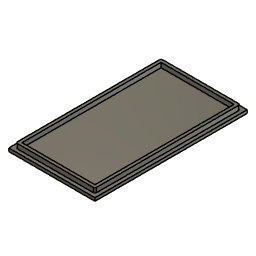
Tapa4_Base Final (Autodesk Fusion 360 design; units mm, degrees)
Autodesk Fusion 360 part; units mm, degrees
sketch "Boceto1" plane through (0, 0, 0) normal (0, 1, 0) x (1, 0, 0)
  line L0 (0, 0) -> (56, 0)
  line L1 (56, 0) -> (56, 99)
  line L2 (56, 99) -> (0, 99)
  line L3 (0, 99) -> (0, 0)
  dimension "d1" = 99
  dimension "d2" = 56
  constraint horizontal L0
  constraint vertical L1
  constraint horizontal L2
  constraint vertical L3
  constraint coincident L0.start L3.end
  measures "d1" distance of L0.start L2.end
  measures "d2" distance of L0.start L0.end
extrude "Extruir1" add sketch "Boceto1" along normal blind 2
sketch "Boceto2" plane through (0, 2, 0) normal (0, 1, 0) x (-1, 0, 0)
  line L0 (0, -99) -> (0, 0)
  line L1 (0, 0) -> (-56, 0)
  line L2 (-56, 0) -> (-56, -99)
  line L3 (-56, -99) -> (0, -99)
  line L4 (-2.3, -96.7) -> (-2.3, -2.3)
  line L5 (-2.3, -2.3) -> (-53.7, -2.3)
  line L6 (-53.7, -2.3) -> (-53.7, -96.7)
  line L7 (-53.7, -96.7) -> (-2.3, -96.7)
  line L8 (-4.3, -94.7) -> (-51.7, -94.7)
  line L9 (-51.7, -94.7) -> (-51.7, -4.3)
  line L10 (-51.7, -4.3) -> (-4.3, -4.3)
  line L11 (-4.3, -4.3) -> (-4.3, -94.7)
  dimension "d5" = -2.3
  dimension "d6" = 2
  dimension "d7" = 2
  dimension "d8" = 2
  dimension "d9" = 2
  constraint horizontal L8
  constraint vertical L9
  constraint horizontal L10
  constraint vertical L11
  measures "d6" distance of L6 L9
  measures "d7" distance of L4 L11
  measures "d8" distance of L7 L8
  measures "d9" distance of L5 L10
extrude "Extruir2" add sketch "Boceto2" along normal blind 3 contours L4 L5 L6 L7
fillet "Empalme1" radius 1 4 edges at (2.3, 3.5, -96.7) (53.7, 3.5, -96.7) (53.7, 3.5, -2.3) (2.3, 3.5, -2.3)
